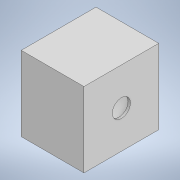
# Autodesk Inventor part: Führung_hochfahren
Saved by Autodesk Inventor 2020.3 (Build 243373000, 373)
## iProperties
Created: 2021-09-30
Part Number: Führung_hochfahren
Material: Generisch
Document SubType Name: Modeling
Designer: Preuß P. Ch.
Density: 1 g/cm^3
Appearance: Vorgabe
Author: Preuß P. Ch.
Autodesk Inventor part; units mm, degrees
ref_plane "YZ Plane" through (0, 0, 0) normal (1, 0, 0) x (0, 1, 0)
ref_plane "XZ Plane" through (0, 0, 0) normal (0, 1, 0) x (-1, 0, 0)
ref_plane "XY Plane" through (0, 0, 0) normal (0, 0, 1) x (1, 0, 0)
sketch "Skizze1" plane through (0, 0, 0) normal (1, 0, 0) x (0, 1, 0)
  line L0 (0, 0) -> (310, 0)
  line L1 (310, 0) -> (310, -310)
  line L2 (310, -310) -> (0, -310)
  line L3 (0, -310) -> (0, 0)
  dimension "d0" = 310
  dimension "d1" = 310
  constraints: 8 end point, 2 parallel, 1 horizontal, 1 perpendicular
  measures "d0" distance of L1.end L2.end
  measures "d1" distance of L0.end L1.end
sketch "Skizze2" plane through (0, 0, 0) normal (1, 0, 0) x (0, 1, 0)
  circle A0 centre (155, -155) radius 105
  point P0 (0, 0)
  dimension "d4" = 210
  constraints: 1 centre point
  measures "d4" diameter of A0
extrude "Extrusion1" add sketch "Skizze1" along normal blind 250
extrude "Extrusion2" cut sketch "Skizze2" along normal blind 250
sketch "Skizze3" plane through (250, 0, 0) normal (1, 0, 0) x (0, 0, -1)
  line L0 (0, 310) -> (0, 0) projected
  line L1 (310, 310) -> (0, 310) projected
  line L2 (0, 0) -> (310, 0)
  line L3 (310, 0) -> (310, 310)
  line L4 (310, 310) -> (0, 310)
  line L5 (0, 310) -> (0, 0)
  constraints: 8 end point, 2 parallel, 1 horizontal, 1 perpendicular
extrude "Extrusion3" add sketch "Skizze3" along normal blind 10
sketch "Skizze4" plane through (260, 0, 0) normal (1, 0, 0) x (0, 0, -1)
  circle A0 centre (155, 155) radius 37.5
  point P0 (0, 0)
  dimension "d13" = 75
  constraints: 1 centre point
  measures "d13" diameter of A0
extrude "Extrusion4" cut sketch "Skizze4" against normal blind 10
sketch "Skizze5" plane through (0, 0, 0) normal (-1, 0, 0) x (0, 0, 1)
  line L0 (-310, 0) -> (-310, 310) projected
  line L1 (-310, 310) -> (-290, 310)
  line L2 (-290, 310) -> (-290, 295)
  line L3 (-290, 295) -> (-310, 295)
  line L4 (-310, 295) -> (-310, 310)
  line L5 (-310, 310) -> (0, 310) projected
  line L6 (0, 310) -> (-20, 310)
  line L7 (-20, 310) -> (-20, 295)
  line L8 (-20, 295) -> (0, 295)
  line L9 (0, 295) -> (0, 310)
  line L10 (0, 0) -> (-310, 0) projected
  line L11 (0, 0) -> (-20, 0)
  line L12 (-20, 0) -> (-20, 15)
  line L13 (-20, 15) -> (0, 15)
  line L14 (0, 15) -> (0, 0)
  line L15 (-310, 0) -> (-290, 0)
  line L16 (-290, 0) -> (-290, 15)
  line L17 (-290, 15) -> (-310, 15)
  line L18 (-310, 15) -> (-310, 0)
  dimension "d16" = 20
  dimension "d17" = 15
  dimension "d18" = 20
  dimension "d19" = 15
  constraints: 32 end point, 8 parallel, 4 horizontal, 4 perpendicular, 4 point on line
  measures "d16" distance of L2.end L3.end
  measures "d17" distance of L1.end L2.end
  measures "d18" distance of L8.end L7.end
  measures "d19" distance of L11.end L12.end
hole "Bohrung1" at (0, 295, -290) at (0, 295, -20) at (0, 15, -20) at (0, 15, -290) direction (1, 0, 0) diameter 8.376 depth 27.3 tip angle 118 thread size "M10x1.5" class "6H" standard "ISO Metric profile"
